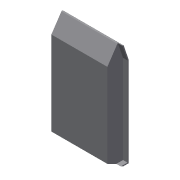
# Autodesk Inventor part: Tank body
Saved by Autodesk Inventor 2015 (Build 190159000, 159)
## iProperties
Created: 2015-03-15
Part Number: Tank body
Material: Generic
Document SubType Name: Modeling
Designer: james_000
Density: 1 g/cm^3
Appearance: Default
Author: james_000
Autodesk Inventor part; units mm, degrees
ref_plane "YZ Plane" through (0, 0, 0) normal (1, 0, 0) x (0, 1, 0)
ref_plane "XZ Plane" through (0, 0, 0) normal (0, 1, 0) x (-1, 0, 0)
ref_plane "XY Plane" through (0, 0, 0) normal (0, 0, 1) x (1, 0, 0)
sketch "Sketch1" plane through (0, 0, 0) normal (1, 0, 0) x (0, 1, 0)
  line L0 (0, 0) -> (0, -150)
  line L1 (20, -160) -> (0, -150)
  line L2 (30, 0) -> (21.3239, 26.0284)
  arc A0 (21.3239, 26.0284) -> (17.6778, 26.5166) centre (19.3814, 25.3809) ccw
  line L3 (0, 0) -> (17.6778, 26.5166)
  line L4 (20, -160) -> (30, -160)
  line L5 (30, -160) -> (30, 0)
  dimension "d0" = 150
  dimension "d4" = 30
  constraints: 12 end point, 2 point on circle, 1 centre point, 1 horizontal, 1 perpendicular, 1 tangent, 1 vertical
  measures "d0" distance of L0.start L0.end
  measures "d4" distance of L0.start L2.start
extrude "Extrusion1" add sketch "Sketch1" along normal blind 100
sketch "Sketch2" plane through (100, 0, 0) normal (1, 0, 0) x (0, 0, -1)
  line L0 (0, 30) -> (160, 30)
  line L1 (160, 30) -> (160, 20)
  line L2 (0, 30) -> (-26.0284, 21.3239)
  line L3 (0, 30) -> (-26.0284, 21.3239) projected
  arc A0 (-26.0284, 21.3239) -> (-26.5166, 17.6778) centre (-25.3809, 19.3814) ccw projected
  arc A1 (-26.0284, 21.3239) -> (-27.3197, 18.7231) centre (-25.3809, 19.3814) ccw
  line L4 (160, 20) -> (160, 30) projected
  line L5 (158, 28) -> (0, 28)
  line L6 (0, 28) -> (-25.3809, 19.3814)
  line L7 (-25.3809, 19.3814) -> (-27.4284, 18.6861)
  line L8 (158, 28) -> (158, 16)
  line L9 (150, 0) -> (160, 20) projected
  line L10 (160, 20) -> (158, 16)
  point P0 (0, 0)
  dimension "d7" = 2
  constraints: 17 end point, 3 point on line, 2 point on circle, 1 centre point, 1 coincident, 1 collinear, 1 horizontal, 1 perpendicular, 1 vertical
  measures "d7" distance of L0.start L5.end
extrude "Extrusion2" add sketch "Sketch2" along normal blind 8
sketch "Sketch3" plane through (0, 30, 0) normal (0, 1, 0) x (1, 0, 0)
  point P0 (0, 0)
body "Solid1"
